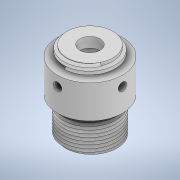
# Autodesk Inventor part: Деталь9
Saved by Autodesk Inventor 2020 (Build 240168000, 168)
## iProperties
Created: 2021-04-26
Part Number: Деталь9
Material: Типовые
Document SubType Name: Modeling
Designer: lbfas
Density: 1 g/cm^3
Appearance: По умолчанию
Author: lbfas
Autodesk Inventor part; units mm, degrees
sketch "Эскиз1" plane through (0, 0, 0) normal (0, 1, 0) x (-1, 0, 0)
  circle A0 centre (0, 0) radius 12.5
  circle A1 centre (0, 0) radius 5.5
  dimension "d0" = 25
  dimension "d1" = 11
  constraints: 2 centre point, 2 coincident
  measures "d0" diameter of A0
  measures "d1" diameter of A1
extrude "Выдавливание1" add sketch "Эскиз1" against normal blind 5.5
sketch "Эскиз2" plane through (0, -5.5, 0) normal (0, -1, 0) x (1, 0, 0)
  circle A0 centre (0, 0) radius 17.75
  circle A1 centre (0, 0) radius 9
  dimension "d4" = 35.5
  dimension "d5" = 18
  constraints: 2 centre point, 2 coincident
  measures "d4" diameter of A0
  measures "d5" diameter of A1
extrude "Выдавливание2" add sketch "Эскиз2" along normal blind 18
sketch "Эскиз3" plane through (0, -23.5, 0) normal (0, -1, 0) x (1, 0, 0)
  circle A0 centre (0, 0) radius 14.5
  circle A1 centre (0, 0) radius 9
  dimension "d8" = 29
  constraints: 2 centre point, 2 coincident
  measures "d8" diameter of A0
extrude "Выдавливание3" add sketch "Эскиз3" along normal blind 18.5
ref_plane "РабПлоскость1" through (0, -11, 0) normal (0, 1, 0) x (1, 0, 0)
sketch "Эскиз4" plane through (0, -11, 0) normal (0, 1, 0) x (1, 0, 0)
  line L0 (0, 0) -> (0, 17.75)
  circle A0 centre (0, 0) radius 17.75 projected
  constraints: 2 end point, 1 vertical, 1 vertical alignment, 1 other
ref_plane "РабПлоскость2" through (0, -11, -17.75) normal (0, 0, -1) x (-1, 0, 0)
sketch "Эскиз5" plane through (0, -11, -17.75) normal (0, 0, -1) x (-1, 0, 0)
  circle A0 centre (0, 0) radius 2.25
  point P0 (0, 11)
  dimension "d12" = 4.5
  constraints: 1 centre point
  measures "d12" diameter of A0
extrude "Выдавливание4" cut sketch "Эскиз5" against normal blind 12.5
pattern_circular "Круговой массив1" count 4 over 360 about axis through (0, -5.5, 0) along (0, -1, 0) of "Выдавливание4"
ref_plane "РабПлоскость3" through (0, -5.5, 0) normal (1, 0, 0) x (0, -1, 0)
sketch "Эскиз7" plane through (0, -5.5, 0) normal (1, 0, 0) x (0, -1, 0)
  line L0 (18.8657, -14.5) -> (18.8657, -13)
  line L1 (18.8657, -13) -> (19.7317, -14.5)
  line L2 (18.8657, -14.5) -> (19.7317, -14.5)
  line L3 (18.8657, -13) -> (17.9997, -14.5)
  line L4 (18.8657, -14.5) -> (17.9997, -14.5)
  line L5 (18, -17.75) -> (18, 17.75) projected
  line L6 (18, -17.75) -> (18, -14.5)
  point P0 (-5.5, 0)
  dimension "d23" = 30
  constraints: 12 end point, 1 horizontal, 1 vertical
  measures "d23" angle of L0 L1
coil "Пружина1" sketch "Эскиз7" operation cut axis through (0, -5.5, 0) along (0, -1, 0) pitch 1.732 turns 11.547344 hand right
sketch "Эскиз8" plane through (0, -5.5, 0) normal (1, 0, 0) x (0, -1, 0)
  line L0 (0, -12.5) -> (0, 12.5) projected
  line L1 (-0.8657, -12.5) -> (0.0003, -12.5)
  line L2 (-0.8657, -12.5) -> (-1.7317, -12.5)
  line L3 (-0.8657, -12.5) -> (-0.8657, -14)
  line L4 (-0.8657, -14) -> (0.0003, -12.5)
  line L5 (-0.8657, -14) -> (-1.7317, -12.5)
  line L6 (-5.5, 12.5) -> (-5.5, -12.5) projected
  line L7 (-1.7317, -12.5) -> (-5.5, -12.5)
  line L8 (-5.5, -12.5) -> (0, -12.5) projected
  point P0 (-5.5, 0)
  dimension "d43" = 3.7683
  constraints: 12 end point, 1 collinear, 1 horizontal
  measures "d43" distance of L2.end L6.end
coil "Пружина2" sketch "Эскиз8" operation add axis through (0, -5.5, 0) along (0, 1, 0) pitch 1.732 turns 2.17552 hand right
sketch "Эскиз9" plane through (0, -5.5, 0) normal (0, 1, 0) x (1, 0, 0)
  point P0 (0, 0)
